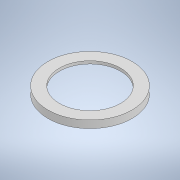
# Autodesk Inventor part: upevnovac_veze
Saved by Autodesk Inventor 2022 (Build 260153000, 153)
## iProperties
Created: 2022-12-19
Part Number: upevnovac_veze
Material: Generic
Document SubType Name: Modeling
Designer: matys
Density: 1 g/cm^3
Appearance: Default
Author: matys
Autodesk Inventor part; units mm, degrees
ref_plane "YZ Plane" through (0, 0, 0) normal (1, 0, 0) x (0, 1, 0)
ref_plane "XZ Plane" through (0, 0, 0) normal (0, 1, 0) x (-1, 0, 0)
ref_plane "XY Plane" through (0, 0, 0) normal (0, 0, 1) x (1, 0, 0)
sketch "Sketch1" plane through (0, 0, 0) normal (0, 1, 0) x (-1, 0, 0)
  circle A0 centre (0, 0) radius 41.5
  line L0 (0, -41.5) -> (0, -45.3)
  circle A1 centre (0, 0) radius 45.3
  dimension "d1" = 83
  dimension "d2" = 3.8
  constraints: 2 coincident, 2 end point, 2 vertical alignment, 1 vertical, 4 other
  measures "d2" distance of L0.start L0.end
extrude "Extrusion1" add sketch "Sketch1" along normal blind 5
sketch "Sketch2" plane through (0, 5, 0) normal (0, 1, 0) x (1, 0, 0)
  circle A0 centre (0, 0) radius 45.3
  circle A1 centre (0, 0) radius 41.5 projected
  line L0 (0, -41.5) -> (0, -33)
  circle A2 centre (0, 0) radius 33
  dimension "d5" = 8.5
  constraints: 2 coincident, 2 end point, 2 vertical alignment, 1 centre point, 1 vertical, 3 other
  measures "d5" distance of L0.start L0.end
extrude "Extrusion2" add sketch "Sketch2" along normal blind 3 contours A0 | A1
body "Solid1"
